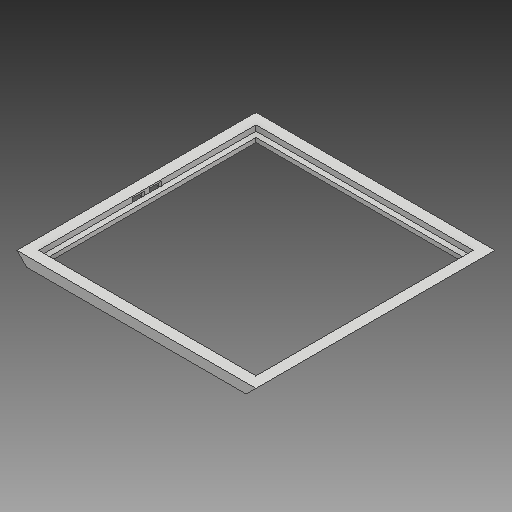
# Autodesk Inventor part: PV_Ramen_CPY_3_CPY
Saved by Autodesk Inventor 2018.3 (Build 223284000, 284)
## iProperties
Created: 2019-09-06
Part Number: PV_Ramen_CPY_3_CPY
Material: Generisch
Document SubType Name: Modeling
Designer: DerLobre
Density: 1 g/cm^3
Appearance: Vorgabe
Author: DerLobre
Autodesk Inventor part; units mm, degrees
ref_plane "YZ Plane" through (0, 0, 0) normal (1, 0, 0) x (0, 1, 0)
sketch "Skizze1" plane through (0, 0, 0) normal (0, 0, 1) x (1, 0, 0)
  line L0 (-220, -220) -> (220, -220) projected
  line L1 (220, 220) -> (220, -220) projected
  line L2 (-220, 220) -> (-220, -220) projected
  line L3 (-220, 220) -> (220, 220) projected
  line L4 (200, 200) -> (-200, 200) projected
  line L5 (-200, 200) -> (-200, -200) projected
  line L6 (-200, -200) -> (200, -200) projected
  line L7 (200, -200) -> (200, 200) projected
  line L8 (220, -220) -> (-220, -220)
  line L9 (-220, -220) -> (-220, 220)
  line L10 (-220, 220) -> (220, 220)
  line L11 (220, 220) -> (220, -220)
  line L12 (200, -200) -> (-200, -200)
  line L13 (-200, -200) -> (-200, 200)
  line L14 (-200, 200) -> (200, 200)
  line L15 (200, 200) -> (200, -200)
  point P0 (0, 0)
  constraints: 16 end point, 4 parallel, 2 horizontal, 2 perpendicular
extrude "Extrusion1" add sketch "Skizze1" against normal blind 18
ref_plane "Arbeitsebene1" through (0, 0, -20) normal (0, 0, 1) x (1, 0, 0)
sketch "Skizze3" plane through (0, 0, -20) normal (0, 0, 1) x (1, 0, 0)
  arc A0 (-205, 25.5) -> (-205, 4.5) centre (-205, 15) ccw projected
  arc A1 (-205, 25.5) -> (-205, 4.5) centre (-205, 15) ccw projected
  arc A2 (-205, -5.9522) -> (-205, -26.9522) centre (-205, -16.4522) ccw projected
  arc A3 (-205, -5.9522) -> (-205, -26.9522) centre (-205, -16.4522) ccw projected
  arc A4 (-205, -5.9522) -> (-205, -26.9522) centre (-205, -16.4522) ccw projected
  arc A5 (-205, -5.9522) -> (-205, -26.9522) centre (-205, -16.4522) ccw projected
  line L0 (-200, -26.9522) -> (-205, -26.9522) projected
  line L1 (-205, -5.9522) -> (-200, -5.9522) projected
  line L2 (-205, 4.5) -> (-200, 4.5)
  line L3 (-200, -200) -> (-200, 200) projected
  line L4 (-205, 25.5) -> (-200, 25.5)
  line L5 (-205, -5.9522) -> (-200, -5.9522)
  line L6 (-205, -26.9522) -> (-200, -26.9522)
  arc A6 (-205, 25.5) -> (-205, 4.5) centre (-205, 15) ccw
  arc A7 (-205, -5.9522) -> (-205, -26.9522) centre (-205, -16.4522) ccw
  point P0 (0, 0)
  constraints: 8 end point, 4 point on circle, 4 tangent, 2 centre point, 2 horizontal, 2 point on line, 1 parallel, 1 perpendicular
extrude "Extrusion2" cut sketch "Skizze3" along normal blind 17
sketch "Skizze5" plane through (0, 0, -20) normal (0, 0, 1) x (1, 0, 0)
  line L0 (-200, -26.9522) -> (-200, -200) projected
  line L1 (-200, -200) -> (200, -200) projected
  line L2 (200, -200) -> (200, 200) projected
  line L3 (-200, 200) -> (200, 200) projected
  line L4 (-200, -200) -> (200, -200)
  line L5 (200, -200) -> (200, 200)
  line L6 (200, 200) -> (-200, 200)
  line L7 (-200, 200) -> (-200, -200)
  line L8 (-190, -190) -> (190, -190)
  line L9 (190, -190) -> (190, 190)
  line L10 (190, 190) -> (-190, 190)
  line L11 (-190, 190) -> (-190, -190)
  point P0 (0, 0)
  dimension "d8" = 10
  dimension "d9" = 10
  dimension "d10" = 10
  dimension "d11" = 10
  constraints: 16 end point, 4 parallel, 2 horizontal, 2 perpendicular
  measures "d8" distance between parallel lines of L0 L11
  measures "d9" distance between parallel lines of L1 L8
  measures "d10" distance between parallel lines of L2 L9
  measures "d11" distance between parallel lines of L10 L3
extrude "Extrusion3" add sketch "Skizze5" along normal blind 8
ref_plane "Arbeitsebene3" through (220, -220, -440) normal (-1, 0, 0) x (0, 0, 1)
sketch "Skizze6" plane through (220, -220, -440) normal (-1, 0, 0) x (0, 0, 1)
  arc A0 (425, 193.0478) -> (425, 214.0478) centre (425, 203.5478) ccw projected
  arc A1 (425, 224.5) -> (425, 245.5) centre (425, 235) ccw projected
  line L0 (425, 224.5) -> (422, 224.5) projected
  line L1 (422, 214.0478) -> (425, 214.0478) projected
  line L2 (425, 193.0478) -> (422, 193.0478) projected
  line L3 (422, 245.5) -> (425, 245.5) projected
  line L4 (422, 193.0478) -> (428, 193.0478) projected
  line L5 (422, 193.0478) -> (425, 193.0478)
  line L6 (422, 214.0478) -> (425, 214.0478)
  line L7 (428, 214.0478) -> (422, 214.0478) projected
  line L8 (420, 245.5) -> (420, 224.5) projected
  line L9 (422, 224.5) -> (425, 224.5)
  line L10 (422, 245.5) -> (425, 245.5)
  line L11 (420, 193.0478) -> (420, 20) projected
  line L12 (422, 193.0478) -> (422, 214.0478)
  line L13 (422, 224.5) -> (422, 245.5)
  arc A2 (425, 193.0478) -> (425, 214.0478) centre (425, 203.5478) ccw
  arc A3 (425, 224.5) -> (425, 245.5) centre (425, 235) ccw
  point P0 (440, 220)
  point P1 (420, 20)
  constraints: 12 end point, 6 point on circle, 3 tangent, 2 centre point, 2 vertical, 1 collinear, 1 midpoint, 1 parallel, 1 perpendicular
extrude "Extrusion4" cut sketch "Skizze6" along normal blind 25
sketch "Skizze7" plane through (0, 0, -20) normal (0, 0, -1) x (-1, 0, 0)
  line L0 (190, 190) -> (190, -190) projected
  line L1 (190, -190) -> (-190, -190) projected
  line L2 (-190, -190) -> (-190, 190) projected
  line L3 (-190, 190) -> (190, 190) projected
  line L4 (200, -200) -> (-200, -200) projected
  line L5 (200, 200) -> (200, -200) projected
  line L6 (-200, 200) -> (200, 200) projected
  line L7 (-200, -200) -> (-200, 200) projected
  line L8 (-200, 200) -> (200, 200) projected
  line L9 (-190, -190) -> (-190, 190) projected
  point P0 (0, 0)
extrude "Extrusion5" cut sketch "Skizze7" against normal blind 2
sketch "Skizze8" plane through (0, 0, -12) normal (0, 0, 1) x (1, 0, 0)
  line L0 (-200, -200) -> (200, -200) projected
  line L1 (200, -200) -> (200, 200) projected
  line L2 (200, 200) -> (-200, 200) projected
  line L3 (-200, 200) -> (-200, -200) projected
  line L4 (190, -190) -> (-190, -190) projected
  line L5 (-190, -190) -> (-190, 190) projected
  line L6 (-190, 190) -> (190, 190) projected
  line L7 (190, 190) -> (190, -190) projected
  line L8 (-200, -200) -> (200, -200) projected
  line L9 (200, -200) -> (200, 200) projected
  line L10 (200, 200) -> (-200, 200) projected
  line L11 (-200, 200) -> (-200, -200) projected
  point P0 (0, 0)
extrude "Extrusion6" add sketch "Skizze8" along normal blind 2
chamfer "Fase2" distance 18 angle 45 5 edges at (220, 122.75, -18) (220, -123.4761, -18) (220, -0.7261, -18) (0, 220, -18) (-220, 0, -18)
